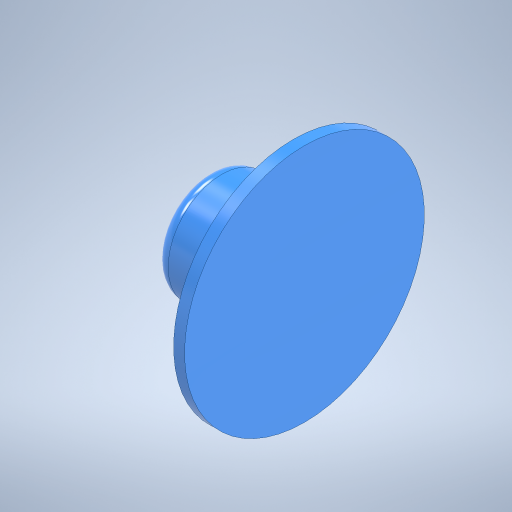
# Autodesk Inventor part: prop_speaker
Saved by Autodesk Inventor 2024.2 (Build 282272000, 272)
## iProperties
Created: 2025-03-01
Part Number: prop_speaker
Material: Všeobecné
Document SubType Name: Modeling
Designer: hepma_axt67em
Density: 1 g/cm^3
Appearance: Světle modrá
Author: hepma_axt67em
Autodesk Inventor part; units mm, degrees
ref_plane "YZ Plane" through (0, 0, 0) normal (1, 0, 0) x (0, 1, 0)
ref_plane "XZ Plane" through (0, 0, 0) normal (0, 1, 0) x (-1, 0, 0)
ref_plane "XY Plane" through (0, 0, 0) normal (0, 0, 1) x (1, 0, 0)
sketch "Náčrt1" plane through (0, 0, 0) normal (0, 0, 1) x (1, 0, 0)
  line L0 (0, 30.12) -> (0, -5.02) projected
  line L1 (-14.21, 0) -> (14.21, 0) projected
  line L2 (10.15, 0) -> (10.15, 25.1)
  line L3 (10.15, 25.1) -> (7.85, 25.1)
  line L4 (7.85, 25.1) -> (7.85, 22)
  line L5 (7.85, 22) -> (6.15, 22)
  line L6 (2.85, 11.25) -> (-10.15, 11.25)
  line L7 (-10.15, 11.25) -> (-10.15, 0)
  line L8 (-10.15, 0) -> (10.15, 0)
  line L9 (4.45, 14) -> (2.85, 14)
  line L10 (2.85, 11.25) -> (2.85, 14)
  line L11 (4.45, 14) -> (4.45, 17)
  line L12 (4.45, 17) -> (6.15, 22)
  point P0 (0, 0)
  point P1 (-10.15, 0)
  dimension "d0" = 25.1
  dimension "d1" = 11.25
  dimension "d2" = 22
  dimension "d3" = 14
  dimension "d4" = 13
  dimension "d5" = 20.3
  dimension "d6" = 3
  dimension "d7" = 2.3
  dimension "d8" = 5.7
  dimension "d9" = 4
  constraints: 22 end point, 6 perpendicular, 2 vertical, 1 collinear, 1 horizontal, 1 parallel, 1 other
  measures "d0" distance of L2.start L2.end
  measures "d1" distance between parallel lines of L1 L6
  measures "d2" distance between parallel lines of L1 L5
  measures "d3" distance between parallel lines of L1 L9
  measures "d4" distance of L6.start L6.end
  measures "d5" distance between parallel lines of L2 L7
  measures "d6" distance of L9.start L11.end
  measures "d7" distance of L2.end L3.end
  measures "d8" distance between parallel lines of L2 L11
  measures "d9" distance from line of L2 L5.end
revolve "Rotace1" add sketch "Náčrt1" angle 360 about axis through (0, 0, 0) along (1, 0, 0)
fillet "Zaoblení1" radius 3 1 edges at (-10.15, -11.25, 0)
